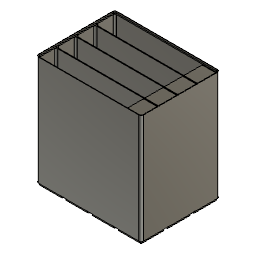
CableBin4x3x25 (Autodesk Fusion 360 design; units mm, degrees)
part number: 2026-05-08-16-53-46-434
Autodesk Fusion 360 part; units mm, degrees
ref_plane "WorkPlane1" through (0, 0, 0) normal (0, 0, 1) x (1, 0, 0)
sketch "Base plate sketch" plane through (0, 0, 0) normal (0, 0, 1) x (1, 0, 0)
  line L0 (-0.25, -0.25) -> (41.75, -0.25)
  line L1 (41.75, -0.25) -> (41.75, 41.75)
  line L2 (41.75, 41.75) -> (-0.25, 41.75)
  line L3 (-0.25, 41.75) -> (-0.25, -0.25)
  dimension "d2" = 0.25
  dimension "d3" = 0.25
  dimension "d4" = 42
  dimension "d5" = 42
  constraint horizontal L0
  constraint vertical L1
  constraint horizontal L2
  constraint vertical L3
  measures "d2" vertical distance of origin L0.start
  measures "d3" horizontal distance of origin L2.end
  measures "d4" horizontal distance of L0.start L0.end
  measures "d5" vertical distance of L0.end L1.end
extrude "Base top section extrude" add sketch "Base plate sketch" against normal blind 2.4 makes body 1
fillet "Base corner fillet" radius 4 8 edges at (-0.25, -0.25, -1.2) (41.75, -0.25, -1.2) (41.75, -0.25, -1.2) (41.75, 41.75, -1.2) (41.75, 41.75, -1.2) (-0.25, 41.75, -1.2) (-0.25, 41.75, -1.2) (-0.25, -0.25, -1.2) on bodies 1
chamfer "Chamfer1" distance 2.4 angle 45 8 edges at (0.9216, 40.5784, -2.4) (-0.25, 20.75, -2.4) (0.9216, 0.9216, -2.4) (20.75, -0.25, -2.4) (40.5784, 0.9216, -2.4) (41.75, 20.75, -2.4) (40.5784, 40.5784, -2.4) (20.75, 41.75, -2.4) on bodies 1
extrude "Extrude2" add 1 faces at (15.6168, 15.0833, -2.4) along direction (0, 0, -1) blind 2.6 on bodies 1 bodies 1
chamfer "Chamfer2" distance 0.8 angle 45 8 edges at (2.6186, 38.8814, -5) (20.75, 39.35, -5) (38.8814, 38.8814, -5) (39.35, 20.75, -5) (38.8814, 2.6186, -5) (20.75, 2.15, -5) (2.6186, 2.6186, -5) (2.15, 20.75, -5) on bodies 1
pattern_linear "R-Pattern1" count 4 spacing 42 along (1, 0, 0) count 3 spacing 42 along (0, 1, 0) of bodies 1 makes body 2 at (68.4167, 16.4167, 0) makes body 3 at (110.4167, 16.4167, 0) makes body 4 at (153.75, 15.0833, 0) makes body 5 at (26.4167, 55.75, 0) makes body 6 at (54.4167, 55.75, 0) makes body 7 at (96.4167, 55.75, 0) makes body 8 at (141.0833, 69.75, 0) makes body 9 at (26.4167, 97.75, 0) makes body 10 at (54.4167, 97.75, 0) makes body 11 at (96.4167, 97.75, 0) makes body 12 at (141.0833, 111.75, 0)
sketch "Simple box sketch" plane through (0, 0, 0) normal (0, 0, 1) x (1, 0, 0)
  line L0 (0, 0) -> (167.5, 0)
  line L1 (167.5, 0) -> (167.5, 125.5)
  line L2 (167.5, 125.5) -> (0, 125.5)
  line L3 (0, 125.5) -> (0, 0)
  dimension "d18" = 167.5
  dimension "d19" = 125.5
  constraint horizontal L0
  constraint vertical L1
  constraint horizontal L2
  constraint vertical L3
  constraint coincident L0.start L3
  constraint coincident L3.end L0
  measures "d18" horizontal distance of L0.start L0.end
  measures "d19" vertical distance of L0.end L1.end
extrude "Simple box extrude" add sketch "Simple box sketch" along normal blind 170 separate body makes body 13
fillet "Bin body corner fillets" radius 3.75 8 edges at (167.5, 125.5, 85) (167.5, 0, 85) (0, 125.5, 85) (167.5, 125.5, 85) (0, 0, 85) (0, 125.5, 85) (167.5, 0, 85) (0, 0, 85) on bodies 13
ref_plane "WorkPlane2" through (0, 0, 170) normal (0, 0, 1) x (1, 0, 0)
sketch "Simple box at point sketch" plane through (0, 0, 170) normal (0, 0, 1) x (1, 0, 0)
  line L0 (0, 0) -> (167.5, 0)
  line L1 (167.5, 0) -> (167.5, 125.5)
  line L2 (167.5, 125.5) -> (0, 125.5)
  line L3 (0, 125.5) -> (0, 0)
  dimension "d25" = 167.5
  dimension "d26" = 125.5
  constraint horizontal L0
  constraint vertical L1
  constraint horizontal L2
  constraint vertical L3
  constraint coincident L0.start L3
  constraint coincident L3.end L0
  measures "d25" horizontal distance of L0.start L0.end
  measures "d26" vertical distance of L0.end L1.end
extrude "Simple box at point extrude" add sketch "Simple box at point sketch" along normal blind 4.4 separate body makes body 14
fillet "Lip body corner fillets" radius 3.75 8 edges at (0, 125.5, 172.2) (167.5, 125.5, 172.2) (167.5, 125.5, 172.2) (167.5, 0, 172.2) (167.5, 0, 172.2) (0, 0, 172.2) (0, 0, 172.2) (0, 125.5, 172.2) on bodies 14
ref_plane "WorkPlane3" through (0, 0, 175) normal (0, 0, 1) x (1, 0, 0)
sketch "Base plate sketch (1)" plane through (0, 0, 175) normal (0, 0, 1) x (1, 0, 0)
  line L0 (-0.5, -0.5) -> (168, -0.5)
  line L1 (168, -0.5) -> (168, 126)
  line L2 (168, 126) -> (-0.5, 126)
  line L3 (-0.5, 126) -> (-0.5, -0.5)
  dimension "d32" = 0.5
  dimension "d33" = 0.5
  dimension "d34" = 168.5
  dimension "d35" = 126.5
  constraint horizontal L0
  constraint vertical L1
  constraint horizontal L2
  constraint vertical L3
  measures "d32" vertical distance of origin L0.start
  measures "d33" horizontal distance of origin L2.end
  measures "d34" horizontal distance of L0.start L0.end
  measures "d35" vertical distance of L0.end L1.end
extrude "Base top section extrude (1)" add sketch "Base plate sketch (1)" against normal blind 2.4 separate body makes body 15
fillet "Base corner fillet (1)" radius 4.25 8 edges at (-0.5, -0.5, 173.8) (168, -0.5, 173.8) (168, -0.5, 173.8) (168, 126, 173.8) (168, 126, 173.8) (-0.5, 126, 173.8) (-0.5, 126, 173.8) (-0.5, -0.5, 173.8) on bodies 15
chamfer "Chamfer3" distance 2.4 angle 45 8 edges at (0.7448, 124.7552, 172.6) (-0.5, 62.75, 172.6) (0.7448, 0.7448, 172.6) (83.75, -0.5, 172.6) (166.7552, 0.7448, 172.6) (168, 62.75, 172.6) (166.7552, 124.7552, 172.6) (83.75, 126, 172.6) on bodies 15
extrude "Extrude6" add 1 faces at (110.4167, 83.0335, 172.6) along direction (0, 0, -1) blind 2.6 on bodies 15 bodies 15
ref_plane "WorkPlane4" through (83.75, 62.75, 174.4) normal (0, 0, 1) x (1, 0, 0)
sketch "Lip top chamfer" plane through (0, 0, 174.4) normal (0, 0, 1) x (1, 0, 0)
  line L0 (0, 0) -> (167.5, 0)
  line L1 (167.5, 0) -> (167.5, 125.5)
  line L2 (167.5, 125.5) -> (0, 125.5)
  line L3 (0, 125.5) -> (0, 0)
  dimension "d44" = 167.5
  dimension "d45" = 125.5
  constraint horizontal L0
  constraint vertical L1
  constraint horizontal L2
  constraint vertical L3
  constraint coincident L0.start L3
  constraint coincident L3.end L0
  measures "d44" horizontal distance of L0.start L0.end
  measures "d45" vertical distance of L0.end L1.end
extrude "Lip top chamfer cut" add sketch "Lip top chamfer" against normal blind 0.6 separate body makes body 16
combine "Combine1" operation cut target body 14 tool bodies 16 15
ref_plane "WorkPlane5" through (0, 0, 170) normal (0, 0, 1) x (1, 0, 0)
sketch "Simple box at point sketch (1)" plane through (0, 0, 170) normal (0, 0, 1) x (1, 0, 0)
  line L0 (1.2, 1.2) -> (166.3, 1.2)
  line L1 (166.3, 1.2) -> (166.3, 124.3)
  line L2 (166.3, 124.3) -> (1.2, 124.3)
  line L3 (1.2, 124.3) -> (1.2, 1.2)
  dimension "d49" = 1.2
  dimension "d50" = 1.2
  dimension "d51" = 165.1
  dimension "d52" = 123.1
  constraint horizontal L0
  constraint vertical L1
  constraint horizontal L2
  constraint vertical L3
  measures "d49" vertical distance of origin L0.start
  measures "d50" horizontal distance of origin L2.end
  measures "d51" horizontal distance of L0.start L0.end
  measures "d52" vertical distance of L0.end L1.end
extrude "Lip bottom chamfer extrude" add sketch "Simple box at point sketch (1)" along normal blind 2.55 separate body makes body 17
fillet "Fillet5" radius 2.55 8 edges at (1.2, 124.3, 171.275) (166.3, 124.3, 171.275) (166.3, 1.2, 171.275) (1.2, 1.2, 171.275) (166.3, 124.3, 171.275) (166.3, 1.2, 171.275) (1.2, 1.2, 171.275) (1.2, 124.3, 171.275) on bodies 17
chamfer "Chamfer4" distance 2.55 angle 45 8 edges at (1.9469, 1.9469, 172.55) (83.75, 1.2, 172.55) (165.5531, 1.9469, 172.55) (166.3, 62.75, 172.55) (165.5531, 123.5531, 172.55) (83.75, 124.3, 172.55) (1.9469, 123.5531, 172.55) (1.2, 62.75, 172.55) on bodies 17
combine "Combine2" operation cut target body 14 tool bodies 17
ref_plane "WorkPlane6" through (0, 0, 170) normal (0, 0, 1) x (1, 0, 0)
sketch "Inner cutout sketch" plane through (0, 0, 170) normal (0, 0, 1) x (1, 0, 0)
  line L0 (1.2, 1.2) -> (166.3, 1.2)
  line L1 (166.3, 1.2) -> (166.3, 31.075)
  line L2 (166.3, 31.075) -> (1.2, 31.075)
  line L3 (1.2, 31.075) -> (1.2, 1.2)
  dimension "d59" = 1.2
  dimension "d60" = 1.2
  dimension "d61" = 165.1
  dimension "d62" = 29.875
  constraint horizontal L0
  constraint vertical L1
  constraint horizontal L2
  constraint vertical L3
  measures "d59" vertical distance of origin L0.start
  measures "d60" horizontal distance of origin L2.end
  measures "d61" horizontal distance of L0.start L0.end
  measures "d62" vertical distance of L0.end L1.end
extrude "Inner cutout extrude" add sketch "Inner cutout sketch" against normal blind 169 separate body makes body 18
fillet "Fillet6" radius 2.55 8 edges at (1.2, 1.2, 85.5) (166.3, 1.2, 85.5) (166.3, 1.2, 85.5) (166.3, 31.075, 85.5) (166.3, 31.075, 85.5) (1.2, 31.075, 85.5) (1.2, 31.075, 85.5) (1.2, 1.2, 85.5) on bodies 18
fillet "Fillet7" radius 2.55 8 edges at (83.75, 31.075, 1) (165.5531, 30.3281, 1) (166.3, 16.1375, 1) (165.5531, 1.9469, 1) (83.75, 1.2, 1) (1.9469, 1.9469, 1) (1.2, 16.1375, 1) (1.9469, 30.3281, 1) on bodies 18
ref_plane "WorkPlane7" through (0, 0, 170) normal (0, 0, 1) x (1, 0, 0)
sketch "Inner cutout sketch (1)" plane through (0, 0, 170) normal (0, 0, 1) x (1, 0, 0)
  line L0 (1.2, 32.275) -> (166.3, 32.275)
  line L1 (166.3, 32.275) -> (166.3, 62.15)
  line L2 (166.3, 62.15) -> (1.2, 62.15)
  line L3 (1.2, 62.15) -> (1.2, 32.275)
  dimension "d70" = 32.275
  dimension "d71" = 1.2
  dimension "d72" = 165.1
  dimension "d73" = 29.875
  constraint horizontal L0
  constraint vertical L1
  constraint horizontal L2
  constraint vertical L3
  measures "d70" vertical distance of origin L0.start
  measures "d71" horizontal distance of origin L2.end
  measures "d72" horizontal distance of L0.start L0.end
  measures "d73" vertical distance of L0.end L1.end
extrude "Inner cutout extrude (1)" add sketch "Inner cutout sketch (1)" against normal blind 169 separate body makes body 19
fillet "Fillet8" radius 2.55 8 edges at (1.2, 32.275, 85.5) (166.3, 32.275, 85.5) (166.3, 32.275, 85.5) (166.3, 62.15, 85.5) (166.3, 62.15, 85.5) (1.2, 62.15, 85.5) (1.2, 62.15, 85.5) (1.2, 32.275, 85.5) on bodies 19
fillet "Fillet9" radius 2.55 8 edges at (83.75, 62.15, 1) (165.5531, 61.4031, 1) (166.3, 47.2125, 1) (165.5531, 33.0219, 1) (83.75, 32.275, 1) (1.9469, 33.0219, 1) (1.2, 47.2125, 1) (1.9469, 61.4031, 1) on bodies 19
ref_plane "WorkPlane8" through (0, 0, 170) normal (0, 0, 1) x (1, 0, 0)
sketch "Inner cutout sketch (2)" plane through (0, 0, 170) normal (0, 0, 1) x (1, 0, 0)
  line L0 (1.2, 63.35) -> (166.3, 63.35)
  line L1 (166.3, 63.35) -> (166.3, 93.225)
  line L2 (166.3, 93.225) -> (1.2, 93.225)
  line L3 (1.2, 93.225) -> (1.2, 63.35)
  dimension "d81" = 63.35
  dimension "d82" = 1.2
  dimension "d83" = 165.1
  dimension "d84" = 29.875
  constraint horizontal L0
  constraint vertical L1
  constraint horizontal L2
  constraint vertical L3
  measures "d81" vertical distance of origin L0.start
  measures "d82" horizontal distance of origin L2.end
  measures "d83" horizontal distance of L0.start L0.end
  measures "d84" vertical distance of L0.end L1.end
extrude "Inner cutout extrude (2)" add sketch "Inner cutout sketch (2)" against normal blind 169 separate body makes body 20
fillet "Fillet10" radius 2.55 8 edges at (1.2, 63.35, 85.5) (166.3, 63.35, 85.5) (166.3, 63.35, 85.5) (166.3, 93.225, 85.5) (166.3, 93.225, 85.5) (1.2, 93.225, 85.5) (1.2, 93.225, 85.5) (1.2, 63.35, 85.5) on bodies 20
fillet "Fillet11" radius 2.55 8 edges at (83.75, 93.225, 1) (165.5531, 92.4781, 1) (166.3, 78.2875, 1) (165.5531, 64.0969, 1) (83.75, 63.35, 1) (1.9469, 64.0969, 1) (1.2, 78.2875, 1) (1.9469, 92.4781, 1) on bodies 20
ref_plane "WorkPlane9" through (0, 0, 170) normal (0, 0, 1) x (1, 0, 0)
sketch "Inner cutout sketch (3)" plane through (0, 0, 170) normal (0, 0, 1) x (1, 0, 0)
  line L0 (1.2, 94.425) -> (166.3, 94.425)
  line L1 (166.3, 94.425) -> (166.3, 124.3)
  line L2 (166.3, 124.3) -> (1.2, 124.3)
  line L3 (1.2, 124.3) -> (1.2, 94.425)
  dimension "d92" = 94.425
  dimension "d93" = 1.2
  dimension "d94" = 165.1
  dimension "d95" = 29.875
  constraint horizontal L0
  constraint vertical L1
  constraint horizontal L2
  constraint vertical L3
  measures "d92" vertical distance of origin L0.start
  measures "d93" horizontal distance of origin L2.end
  measures "d94" horizontal distance of L0.start L0.end
  measures "d95" vertical distance of L0.end L1.end
extrude "Inner cutout extrude (3)" add sketch "Inner cutout sketch (3)" against normal blind 169 separate body makes body 21
fillet "Fillet12" radius 2.55 8 edges at (1.2, 94.425, 85.5) (166.3, 94.425, 85.5) (166.3, 94.425, 85.5) (166.3, 124.3, 85.5) (166.3, 124.3, 85.5) (1.2, 124.3, 85.5) (1.2, 124.3, 85.5) (1.2, 94.425, 85.5) on bodies 21
fillet "Fillet13" radius 2.55 8 edges at (83.75, 124.3, 1) (165.5531, 123.5531, 1) (166.3, 109.3625, 1) (165.5531, 95.1719, 1) (83.75, 94.425, 1) (1.9469, 95.1719, 1) (1.2, 109.3625, 1) (1.9469, 123.5531, 1) on bodies 21
ref_plane "WorkPlane10" through (0, 0, 170) normal (0, 0, 1) x (1, 0, 0)
sketch "Inner cutout sketch (4)" plane through (0, 0, 170) normal (0, 0, 1) x (1, 0, 0)
  line L0 (1.2, 1.2) -> (166.3, 1.2)
  line L1 (166.3, 1.2) -> (166.3, 124.3)
  line L2 (166.3, 124.3) -> (1.2, 124.3)
  line L3 (1.2, 124.3) -> (1.2, 1.2)
  dimension "d103" = 1.2
  dimension "d104" = 1.2
  dimension "d105" = 165.1
  dimension "d106" = 123.1
  constraint horizontal L0
  constraint vertical L1
  constraint horizontal L2
  constraint vertical L3
  measures "d103" vertical distance of origin L0.start
  measures "d104" horizontal distance of origin L2.end
  measures "d105" horizontal distance of L0.start L0.end
  measures "d106" vertical distance of L0.end L1.end
extrude "Inner cutout extrude (4)" add sketch "Inner cutout sketch (4)" against normal blind 0.5 separate body makes body 22
fillet "Fillet14" radius 2.55 8 edges at (1.2, 1.2, 169.75) (166.3, 1.2, 169.75) (166.3, 1.2, 169.75) (166.3, 124.3, 169.75) (166.3, 124.3, 169.75) (1.2, 124.3, 169.75) (1.2, 124.3, 169.75) (1.2, 1.2, 169.75) on bodies 22
combine "Combine3" operation cut target body 13 tool bodies 18 19 20 21 22
combine "Combine4" operation add target body 13 tool bodies 14
ref_plane "WorkPlane11" through (0, 0, 0) normal (0, 0, 1) x (1, 0, 0)
sketch "Base clearance cut sketch" plane through (0, 0, 0) normal (0, 0, 1) x (1, 0, 0)
  line L0 (3.75, 0) -> (163.75, 0)
  line L1 (167.5, 3.75) -> (167.5, 121.75)
  line L2 (163.75, 125.5) -> (3.75, 125.5)
  line L3 (0, 121.75) -> (0, 3.75)
  arc A0 (163.75, 0) -> (167.5, 3.75) centre (163.75, 3.75) ccw
  arc A1 (167.5, 121.75) -> (163.75, 125.5) centre (163.75, 121.75) ccw
  arc A2 (3.75, 125.5) -> (0, 121.75) centre (3.75, 121.75) ccw
  arc A3 (0, 3.75) -> (3.75, 0) centre (3.75, 3.75) ccw
  arc A4 (163.75, -10) -> (177.5, 3.75) centre (163.75, 3.75) ccw
  line L4 (177.5, 3.75) -> (177.5, 121.75)
  arc A5 (177.5, 121.75) -> (163.75, 135.5) centre (163.75, 121.75) ccw
  line L5 (163.75, 135.5) -> (3.75, 135.5)
  arc A6 (3.75, 135.5) -> (-10, 121.75) centre (3.75, 121.75) ccw
  line L6 (-10, 121.75) -> (-10, 3.75)
  arc A7 (-10, 3.75) -> (3.75, -10) centre (3.75, 3.75) ccw
  line L7 (3.75, -10) -> (163.75, -10)
  point P0 (167.5, 0)
  point P1 (167.5, 125.5)
  dimension "d112" = 167.5
  dimension "d113" = 125.5
  dimension "d114" = 3.75
  dimension "d115" = 10
  constraint horizontal L0
  constraint vertical L1
  constraint horizontal L2
  constraint vertical L3
  constraint coincident origin L3
  constraint coincident origin L0
  constraint coincident P0 L0
  constraint coincident P0 L1
  constraint tangent L0 A0
  constraint tangent L1 A0
  constraint coincident P1 L1
  constraint coincident P1 L2
  constraint tangent L1 A1
  constraint tangent L2 A1
  constraint tangent L2 A2
  constraint tangent L3 A2
  constraint tangent L3 A3
  constraint tangent L0 A3
  constraint equal A0 A1
  constraint equal A1 A2
  constraint equal A2 A3
  measures "d112" horizontal distance of origin P0
  measures "d113" vertical distance of P0 P1
  measures "d114" radius of A0
extrude "Base side clearance cut" cut sketch "Base clearance cut sketch" along normal blind 1000 and the other way blind 1000 bodies 1 2 3 4 5 6 7 8 9 10 11 12 13
combine "Combine5" operation add target body 13 tool bodies 2 3 4 5 6 7 8 9 10 11 12 1 1
ref_plane "WorkPlane12" through (83.75, 124.3, 86.775) normal (0, -1, 0) x (-1, 0, 0)
sketch "Sketch13" plane through (0, 124.3, 0) normal (0, -1, 0) x (-1, 0, 0)
  line L0 (-140.2389, -168.8071) -> (-166.4179, -168.8071)
  line L1 (-166.4179, -168.8071) -> (-166.4179, -147.6625)
  line L2 (-166.4179, -147.6625) -> (-140.2389, -168.8071)
  constraint horizontal L0
  constraint perpendicular L0 L1
extrude "Extrude15" add sketch "Sketch13" along normal blind 18.299 separate body makes body 23
extrude "Extrude16" add 1 faces at (157.6916, 106.001, 161.7589) along direction (0, -1, 0) blind 104.881 on bodies 23 bodies 13 23
equation "d6 = -( 2.40 mm )"
equation "d36 = -( 2.40 mm )"
equation "d46 = -( 0.60 mm )"
equation "d63 = -( 169.00 mm )"
equation "d74 = -( 169.00 mm )"
equation "d85 = -( 169.00 mm )"
equation "d96 = -( 169.00 mm )"
equation "d107 = -( 0.50 mm )"
named bodies: "Base", "Base (1)", "Base (2)", "Base (3)", "Base (4)", "Base (5)", "Base (6)", "Base (7)", "Base (8)", "Base (9)", "Base (10)", "Base (11)", "Gridfinity bin 3x4x25", "Lip body", "Lip cutout", "Inner cutout", "Inner cutout (1)", "Inner cutout (2)", "Inner cutout (3)", "Inner cutout (4)"
